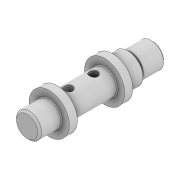
# Autodesk Inventor part: hridel
Saved by Autodesk Inventor 2021 (Build 250183000, 183)
## iProperties
Created: 2021-02-01
Part Number: hridel
Material: Generic
Document SubType Name: Modeling
Designer: adm_topka
Density: 1 g/cm^3
Appearance: Default
Author: adm_topka
Autodesk Inventor part; units mm, degrees
ref_plane "YZ Plane" through (0, 0, 0) normal (1, 0, 0) x (0, 1, 0)
sketch "Sketch1" plane through (0, 0, 0) normal (0, 1, 0) x (-1, 0, 0)
  line L0 (0, 103.1729) -> (0, -96.1307) construction
  line L1 (0, 97.5445) -> (10.5, 97.5445)
  line L2 (10.5, 97.5445) -> (12.5, 95.5445)
  line L3 (12.5, 95.5445) -> (12.5, 75.5445)
  line L4 (12.5, 75.5445) -> (20, 75.5445)
  line L5 (20, 75.5445) -> (20, 67.5445)
  line L6 (20, 67.5445) -> (12.5, 67.5445)
  line L7 (12.5, 67.5445) -> (12.5, 20.5445)
  line L8 (12.5, 20.5445) -> (20, 20.5445)
  line L9 (20, 20.5445) -> (20, 12.5445)
  line L10 (11, -2.4555) -> (11, -5.4555)
  line L11 (11, -5.4555) -> (12.5, -5.4555)
  line L12 (12.5, -5.4555) -> (12.5, -25.4555)
  line L13 (12.5, -25.4555) -> (10.5, -27.4555)
  line L14 (10.5, -27.4555) -> (0, -27.4555)
  line L15 (0, 97.5445) -> (0, -27.4555)
  line L16 (11, -2.4555) -> (15, -2.4555)
  line L17 (15, -2.4555) -> (15, 12.5445)
  line L18 (15, 12.5445) -> (20, 12.5445)
  point P0 (0, 0)
  dimension "d0" = 12.5
  dimension "d1" = 125
  dimension "d2" = 20
  dimension "d3" = 8
  dimension "d4" = 8
  dimension "d5" = 12.5
  dimension "d7" = 3
  dimension "d9" = 2
  dimension "d10" = 135
  dimension "d11" = 2
  dimension "d14" = 15
  dimension "d23" = 95
  dimension "d24" = 40
  dimension "d32" = 25
  constraints: 38 end point, 11 perpendicular, 7 point on line, 2 horizontal, 1 collinear, 1 vertical
  measures "d0" distance between parallel lines of L7 L0
  measures "d1" distance between parallel lines of L14 L1
  measures "d2" distance between parallel lines of L0 L5
  measures "d3" distance of L4.end L5.end
  measures "d4" distance of L8.end L9.end
  measures "d5" distance between parallel lines of L0 L12
  measures "d7" distance of L10.start L10.end
  measures "d9" distance from line of L2.end L1
  measures "d10" angle of L2 L1
  measures "d11" distance from line of L12.end L14
  measures "d14" distance between parallel lines of L0 L17
  measures "d23" distance between parallel lines of L6 L14
  measures "d24" distance between parallel lines of L18 L14
  measures "d32" distance between parallel lines of L14 L16
revolve "Revolution1" add sketch "Sketch1" angle 360 about axis through (0, 0, 103.1729) along (0, 0, -1)
fillet "Fillet1" radius 1 3 edges at (12.5, 0, 75.5445) (12.5, 0, 67.5445) (12.5, 0, 20.5445)
fillet "Fillet2" radius 1 1 edges at (15, 0, 12.5445)
ref_plane "Work Plane1" through (-12.5, 0, -25.4555) normal (-1, 0, 0) x (0, -1, 0)
sketch "Sketch2" plane through (-12.5, 0, -25.4555) normal (-1, 0, 0) x (0, -1, 0)
  line L0 (0, -15) -> (0, 15) construction
  line L1 (-12.5, 0) -> (12.5, 0) projected
  line L2 (3, -15) -> (3, 15)
  line L3 (-3, 15) -> (-3, -15)
  arc A0 (-3, -15) -> (3, -15) centre (0, -15) ccw
  arc A1 (3, 15) -> (-3, 15) centre (0, 15) ccw
  line L4 (-10.5, -2) -> (10.5, -2) projected
  point P0 (0, 25.4555)
  point P1 (0, 0)
  point P2 (-3, -2)
  point P3 (3, -2)
  dimension "d16" = 6
  dimension "d17" = 17
  constraints: 8 end point, 4 point on circle, 4 tangent, 2 centre point, 2 midpoint, 1 parallel, 1 perpendicular
  measures "d16" distance between parallel lines of L2 L3
  measures "d17" distance from line of L4 L2.end
extrude "Extrusion1" cut sketch "Sketch2" against normal blind 4.1 contours L3 A1 L2 L1 | L1 L2 L4 L3
ref_plane "Work Plane2" through (0, 12.5, 0) normal (0, 1, 0) x (-1, 0, 0)
sketch "Sketch5" plane through (0, 12.5, 0) normal (0, 1, 0) x (-1, 0, 0)
  line L0 (-20, 67.5445) -> (20, 67.5445) projected
  line L1 (-20, 20.5445) -> (20, 20.5445) projected
  line L2 (12.5, 66.5445) -> (-12.5, 66.5445) projected
  line L3 (-12.5, 21.5445) -> (12.5, 21.5445) projected
  line L4 (12.5, 66.5445) -> (-12.5, 66.5445) projected
  line L5 (0, 66.5445) -> (0, 21.5445)
  line L6 (-12.5, 21.5445) -> (12.5, 21.5445) projected
  point P0 (0, 0)
  point P1 (0, 56.5445)
  point P2 (0, 31.5445)
  dimension "d21" = 11
  dimension "d22" = 25
  constraints: 2 end point, 2 midpoint, 2 point on line
  measures "d21" distance from line of L0 point (0, 56.545)
  measures "d22" distance of point (0, 31.545) point (0, 56.545)
hole "Hole1" at (0, 12.5, 56.5445) at (0, 12.5, 31.5445) direction (0, -1, 0) diameter 8.376 end through all thread size "M10x1.5" class "6H" standard "ISO Metric profile"
equation "\"d5\" = d0"
body "Solid1"
